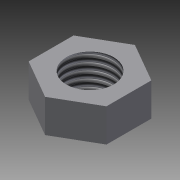
# Autodesk Inventor part: ThreadedBar2
Saved by Autodesk Inventor 2015 (Build 190159000, 159)
## iProperties
Created: 2017-01-04
Part Number: ThreadedBar2
Material: Generic
Document SubType Name: Modeling
Designer: Ernest
Density: 1 g/cm^3
Appearance: Default
Mass: 1.09156 g
Surface Area: 9.30785 cm^2
Volume: 1.09156 cm^3
Author: Ernest
Autodesk Inventor part; units mm, degrees
ref_plane "YZ Plane" through (0, 0, 0) normal (1, 0, 0) x (0, 1, 0)
ref_plane "XZ Plane" through (0, 0, 0) normal (0, 1, 0) x (-1, 0, 0)
ref_plane "XY Plane" through (0, 0, 0) normal (0, 0, 1) x (1, 0, 0)
sketch "Sketch1" plane through (0, 0, 0) normal (0, 0, 1) x (1, 0, 0)
  circle A0 centre (0, 0) radius 5
  line L0 (0, 9.5) -> (8.2272, 4.75)
  line L1 (8.2272, 4.75) -> (8.2272, -4.75)
  line L2 (8.2272, -4.75) -> (0, -9.5)
  line L3 (0, -9.5) -> (-8.2272, -4.75)
  line L4 (-8.2272, -4.75) -> (-8.2272, 4.75)
  line L5 (-8.2272, 4.75) -> (0, 9.5)
  dimension "d0" = 10
  dimension "d7" = 19
  constraints: 12 end point, 2 coincident, 1 centre point, 13 other
  measures "d0" diameter of A0
  measures "d7" distance of L0.start L2.end
extrude "Extrusion1" add sketch "Sketch1" along normal blind 7
thread "Thread2" size "M10x1.5" class "6H" standard "ANSI Metric M Profile" full length
body "Solid1"
